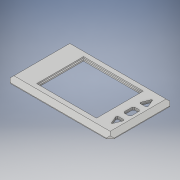
# Autodesk Inventor part: TopCover
Saved by Autodesk Inventor 2019 (Build 230136000, 136)
## iProperties
Created: 2021-04-26
Part Number: TopCover
Material: Všeobecné
Document SubType Name: Modeling
Designer: miko flosso
Density: 1 g/cm^3
Appearance: Výchozí
Author: miko flosso
Autodesk Inventor part; units mm, degrees
ref_plane "YZ Plane" through (0, 0, 0) normal (1, 0, 0) x (0, 1, 0)
ref_plane "XZ Plane" through (0, 0, 0) normal (0, 1, 0) x (-1, 0, 0)
ref_plane "XY Plane" through (0, 0, 0) normal (0, 0, 1) x (1, 0, 0)
sketch "Náčrt1" plane through (0, 0, 0) normal (0, 1, 0) x (-1, 0, 0)
  line L0 (0, 0) -> (-80, 0)
  line L1 (-80, 0) -> (-80, -49)
  line L2 (-80, -49) -> (0, -49)
  line L3 (0, -49) -> (0, 0)
  dimension "d0" = 80
  dimension "d1" = 49
  constraints: 8 end point, 2 parallel, 1 horizontal, 1 perpendicular
  measures "d0" distance of L2.end L1.end
  measures "d1" distance of L1.end L0.end
extrude "Vysunutí1" add sketch "Náčrt1" along normal blind 3.5
chamfer "Zkosení1" distance 3 angle 45 4 edges at (0, 1.75, 0) (0, 1.75, -49) (80, 1.75, -49) (80, 1.75, 0)
chamfer "Zkosení2" distance 3 angle 45 4 edges at (40, 3.5, 0) (0, 3.5, -24.5) (40, 3.5, -49) (80, 3.5, -24.5)
shell "Skořepina1" thickness 2 removed faces 1 at (27.6667, 0, -32.6667)
sketch "Náčrt2" plane through (0, 3.5, 0) normal (0, 1, 0) x (1, 0, 0)
  line L0 (18, 41.5) -> (62, 41.5)
  line L1 (62, 41.5) -> (62, 7.5)
  line L2 (62, 7.5) -> (18, 7.5)
  line L3 (18, 7.5) -> (18, 41.5)
  line L4 (77, 49) -> (3, 49) projected
  line L5 (0, 46) -> (0, 3) projected
  point P0 (0, 0)
  dimension "d11" = 44
  dimension "d12" = 34
  dimension "d13" = 7.5
  dimension "d14" = 18
  constraints: 8 end point, 2 parallel, 1 horizontal, 1 perpendicular
  measures "d11" distance of L1.end L2.end
  measures "d12" distance of L0.end L1.end
  measures "d13" distance between parallel lines of L0 L4
  measures "d14" distance between parallel lines of L3 L5
extrude "Vysunutí2" cut sketch "Náčrt2" against normal blind 2.5
sketch "Náčrt3" plane through (0, 3.5, 0) normal (0, 1, 0) x (1, 0, 0)
  line L0 (63, 42.5) -> (17, 42.5)
  line L1 (17, 42.5) -> (17, 6.5)
  line L2 (17, 6.5) -> (63, 6.5)
  line L3 (63, 6.5) -> (63, 42.5)
  line L4 (63, 42.5) -> (17, 6.5) construction
  line L5 (17, 42.5) -> (63, 6.5) construction
  point P0 (0, 0)
  point P1 (40, 24.5)
  dimension "d17" = 46
  dimension "d18" = 36
  constraints: 12 end point, 2 midpoint, 2 parallel, 1 horizontal, 1 perpendicular
  measures "d17" distance of L2.end L1.end
  measures "d18" distance of L1.end L0.end
extrude "Vysunutí3" cut sketch "Náčrt3" against normal blind 1
sketch "Náčrt4" plane through (0, 3.5, 0) normal (0, 1, 0) x (1, 0, 0)
  line L0 (75.5, 16) -> (69, 16)
  line L1 (69, 16) -> (72.25, 8)
  line L2 (75.5, 16) -> (72.25, 8)
  line L3 (3, 0) -> (77, 0) projected
  line L4 (0, 46) -> (0, 3) projected
  point P0 (0, 0)
  dimension "d21" = 6.5
  constraints: 6 end point
  measures "d21" distance of L0.end L0.start
extrude "Vysunutí4" cut sketch "Náčrt4" against normal blind 2.5
chamfer "Zkosení3" distance 1 angle 45 3 edges at (69, 2.5, -16) (75.5, 2.5, -16) (72.25, 2.5, -8)
ref_plane "Pracovní rovina1" through (77, 0, -24.5) normal (0, 0, -1) x (-1, 0, 0)
mirror "Zrcadlit1" about plane through (77, 0, -24.5) normal (0, 0, -1) of "Vysunutí4", "Zkosení3"
sketch "Náčrt5" plane through (0, 3.5, 0) normal (0, 1, 0) x (1, 0, 0)
  line L0 (69.3705, 20.5) -> (74.8705, 20.5)
  line L1 (74.8705, 20.5) -> (74.8705, 28.5)
  line L2 (74.8705, 28.5) -> (69.3705, 28.5)
  line L3 (69.3705, 28.5) -> (69.3705, 20.5)
  line L4 (3, 0) -> (77, 0) projected
  point P0 (0, 0)
  dimension "d30" = 5.5
  dimension "d31" = 8
  dimension "d32" = 20.5
  constraints: 8 end point, 2 parallel, 1 horizontal, 1 perpendicular
  measures "d30" distance of L2.end L1.end
  measures "d31" distance of L1.end L0.end
  measures "d32" distance between parallel lines of L4 L0
extrude "Vysunutí5" cut sketch "Náčrt5" against normal blind 2.5
chamfer "Zkosení4" distance 1 angle 45 4 edges at (69.3705, 2.5, -28.5) (69.3705, 2.5, -20.5) (74.8705, 2.5, -20.5) (74.8705, 2.5, -28.5)
